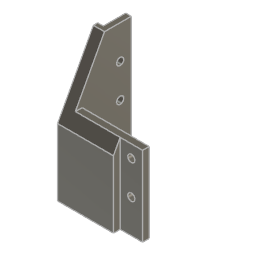
Fender-Front (Autodesk Fusion 360 design; units mm, degrees)
part number: 2026-04-13-00-12-13-494
Autodesk Fusion 360 part; units mm, degrees
sketch "Sketch1" plane through (0, 0, 0) normal (0, 0, 1) x (1, 0, 0)
  line L0 (0, 0) -> (5, 0)
  line L1 (5, 6) -> (5, 18)
  line L2 (2.5, 18) -> (0, 18)
  line L3 (0, 18) -> (0, 0)
  line L4 (5, 6) -> (25, 6)
  line L5 (25, 3) -> (25, 0)
  line L6 (25, 0) -> (5, 0)
  circle A0 centre (2.5, 4.5) radius 1.175
  circle A1 centre (2.5, 13.5) radius 1.175
  circle A2 centre (10, 3) radius 1.425
  circle A3 centre (20, 3) radius 1.425
  line L7 (2.5, 18) -> (2.5, 28)
  line L8 (2.5, 28) -> (5, 28)
  line L9 (5, 28) -> (5, 18)
  line L10 (25, 6) -> (35, 6)
  line L11 (35, 6) -> (35, 3)
  line L12 (35, 3) -> (25, 3)
  dimension "d3" = 2.85
  dimension "d4" = 2.35
  constraint horizontal L0
  constraint vertical L1
  constraint horizontal L2
  constraint vertical L3
  constraint coincident L0.start L3.end
  constraint perpendicular L3 L4
  constraint perpendicular L4 L5
  constraint perpendicular L1 L6
  constraint vertical L7
  constraint horizontal L8
  constraint vertical L9
  constraint perpendicular L5 L10
  constraint perpendicular L10 L11
  constraint perpendicular L5 L12
  measures "d3" diameter of A2
  measures "d4" diameter of A1
extrude "Extrude1" add sketch "Sketch1" along normal blind 60 contours L0 L1 L2 L3 L4 L5 L6 L7 L8 L9 L10 L11 L12 | A0 | A1 | A2 | A3
sketch "Sketch2" plane through (2.5, 0, 0) normal (-1, 0, 0) x (0, -1, 0)
  line L0 (-28, 0) -> (-18, 0)
  line L1 (-18, 0) -> (-18, 60)
  line L2 (-18, 60) -> (-28, 60)
  line L3 (-28, 60) -> (-28, 0)
  circle A0 centre (-23, 30) radius 1.6
  circle A1 centre (-23, 45) radius 1.6
  circle A2 centre (-23, 15) radius 1.6
extrude "Extrude2" cut sketch "Sketch2" against normal blind 2.5 contours A0 | A1 | A2
sketch "Sketch3" plane through (0, 3, 0) normal (0, -1, 0) x (1, 0, 0)
  line L0 (25, 0) -> (35, 0)
  line L1 (35, 0) -> (35, 60)
  line L2 (35, 60) -> (25, 60)
  line L3 (25, 60) -> (25, 0)
  circle A0 centre (30, 30) radius 1.6
  circle A1 centre (30, 15) radius 1.6
extrude "Extrude3" cut sketch "Sketch3" against normal blind 3 contours A0 | A1
sketch "Sketch4" plane through (0, 0, 0) normal (0, 0, -1) x (1, 0, 0)
  line L0 (5, -28) -> (5, -6)
  line L1 (5, -6) -> (35, -6)
  line L2 (35, -6) -> (35, -3)
  line L3 (35, -3) -> (25, -3)
  line L4 (25, -3) -> (25, 0)
  line L5 (25, 0) -> (0, 0)
  line L6 (0, 0) -> (0, -18)
  line L7 (0, -18) -> (2.5, -18)
  line L8 (2.5, -18) -> (2.5, -28)
  line L9 (2.5, -28) -> (5, -28)
  circle A0 centre (20, -3) radius 1.4
  circle A1 centre (10, -3) radius 1.4
  circle A2 centre (2.5, -4.5) radius 1.15
  circle A3 centre (2.5, -13.5) radius 1.15
  dimension "d15" = 2.8
  dimension "d18" = 2.3
  measures "d15" diameter of A0
  measures "d18" diameter of A2
extrude "Extrude4" cut sketch "Sketch4" against normal blind 15 contours A0 | A1 | A2 | A3
sketch "Sketch5" plane through (0, 0, 60) normal (0, 0, 1) x (-1, 0, 0)
  line L0 (-5, -6) -> (-5, -28)
  line L1 (-5, -28) -> (-2.5, -28)
  line L2 (-2.5, -28) -> (-2.5, -18)
  line L3 (-2.5, -18) -> (0, -18)
  line L4 (0, -18) -> (0, 0)
  line L5 (0, 0) -> (-25, 0)
  line L6 (-25, 0) -> (-25, -3)
  line L7 (-25, -3) -> (-35, -3)
  line L8 (-35, -3) -> (-35, -6)
  line L9 (-35, -6) -> (-5, -6)
  circle A0 centre (-2.5, -4.5) radius 1.15
  circle A1 centre (-2.5, -13.5) radius 1.15
  circle A2 centre (-10, -3) radius 1.4
  circle A3 centre (-20, -3) radius 1.4
chamfer "Chamfer2" distance 16 distance2 30 1 edges at (12.5, 0, 60) measured on face at (10, 2, 60)
sketch "Sketch6" plane through (35, 0, 0) normal (1, 0, 0) x (0, 1, 0)
  line L0 (6, 41.25) -> (3, 35.625)
  line L1 (3, 35.625) -> (3, 0)
  line L2 (3, 0) -> (6, 0)
  line L3 (6, 0) -> (6, 41.25)
  line L4 (3, 35.625) -> (6, 35.625)
  constraint coincident L0.end L1.start
  constraint coincident L3 L4.end
  constraint perpendicular L3 L4
extrude "Extrude6" cut sketch "Sketch6" against normal blind 30 contours L0 L3 L4
sketch "Sketch7" plane through (5, 0, 0) normal (1, 0, 0) x (0, 1, 0)
  line L0 (16, 60) -> (3, 35.625)
  line L1 (3, 35.625) -> (6, 35.625)
  line L2 (6, 35.625) -> (6, 0)
  line L3 (6, 0) -> (28, 0)
  line L4 (28, 0) -> (28, 60)
  line L5 (28, 60) -> (16, 60)
  circle A0 centre (23, 15) radius 1.6
  circle A1 centre (23, 30) radius 1.6
  circle A2 centre (23, 45) radius 1.6
  circle A3 centre (13.5, 26) radius 1.35
  dimension "d32" = 2.7
  measures "d32" diameter of A3
extrude "Extrude7" cut sketch "Sketch7" against normal blind 3.5 contours A3
mirror "Mirror1" [rolled back] mirror stitch tolerance 0.1
move_body "Move1" [rolled back]
